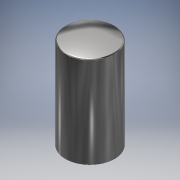
# Autodesk Inventor part: Gondola Pole Caps
Saved by Autodesk Inventor 2018 (Build 220112000, 112)
## iProperties
Created: 2018-02-09
Part Number: Gondola Pole Caps
Material: Steel, Alloy
Document SubType Name: Modeling
Designer: Joey
Density: 7.73 g/cm^3
Appearance: Semi-Polished
Author: Joey
Autodesk Inventor part; units mm, degrees
ref_plane "YZ Plane" through (0, 0, 0) normal (1, 0, 0) x (0, 1, 0)
ref_plane "XZ Plane" through (0, 0, 0) normal (0, 1, 0) x (-1, 0, 0)
ref_plane "XY Plane" through (0, 0, 0) normal (0, 0, 1) x (1, 0, 0)
sketch "Sketch1" plane through (0, 0, 0) normal (0, 0, 1) x (1, 0, 0)
  line L0 (31.75, 0) -> (31.75, 152.4)
  line L1 (31.75, 152.4) -> (0, 152.4)
  line L2 (-31.75, 152.4) -> (-31.75, 0)
  line L3 (-31.75, 0) -> (-44.45, 0)
  line L4 (-44.45, 0) -> (-44.45, 165.1)
  line L5 (-44.45, 165.1) -> (19.05, 165.1)
  line L6 (44.45, 165.1) -> (44.45, 0)
  line L7 (44.45, 0) -> (31.75, 0)
  line L8 (0, 152.4) -> (0, 0) construction
  line L9 (0, 0) -> (76.8208, 0) construction
  arc A0 (44.45, 165.1) -> (0, 171.7263) centre (0, 19.3263) ccw
  arc A1 (0, 171.7263) -> (-44.45, 165.1) centre (0, 19.3263) ccw
  line L10 (19.05, 165.1) -> (44.45, 165.1)
  line L11 (0, 152.4) -> (-31.75, 152.4)
  line L12 (0, 171.7263) -> (0, 152.4)
  dimension "d0" = 152.4
  dimension "d2" = 12.7
  dimension "d4" = 12.7
  dimension "d5" = 152.4
  dimension "d8" = 63.5
  constraints: 26 end point, 11 perpendicular, 4 point on circle, 3 vertical, 2 centre point, 2 point on line, 1 collinear, 1 horizontal, 1 other
  measures "d0" distance of L0.start L0.end
  measures "d2" distance of L2.end L3.end
  measures "d4" distance between parallel lines of L1 L5
  measures "d5" radius of A0
  measures "d8" distance between parallel lines of L0 L2
revolve "Revolution1" add sketch "Sketch1" angle 360 about axis through (0, 152.4, 0) along (0, -1, 0) contours L0 L1 L12 L5 L10 L6 L7 | L10 L5 L12 A0
fillet "Fillet1" radius 3.175 1 edges at (-44.45, 165.1, 0)
body "Solid1"
